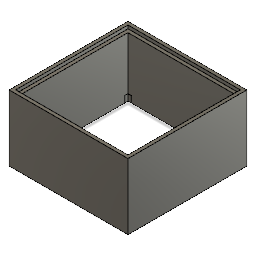
Body-bottom (Autodesk Fusion 360 design; units mm, degrees)
Autodesk Fusion 360 part; units mm, degrees
sketch "Sketch2" plane through (0, 0, 0) normal (0, 1, 0) x (1, 0, 0)
  line L0 (-80, -90) -> (100, -90)
  line L1 (100, -90) -> (100, 90)
  line L2 (100, 90) -> (-80, 90)
  line L3 (-80, 90) -> (-80, -90)
  dimension "d3" = 180
  dimension "d4" = 180
  constraint horizontal L0
  constraint vertical L1
  constraint horizontal L2
  constraint vertical L3
  measures "d3" distance of L0.start L0.end
  measures "d4" distance of L0.start L2.end
extrude "Extrude1" add sketch "Sketch2" along normal blind 100
sketch "Sketch3" plane through (0, 100, 0) normal (0, 1, 0) x (-1, 0, 0)
  line L0 (80, -90) -> (80, 90)
  line L1 (80, 90) -> (-100, 90)
  line L2 (-100, 90) -> (-100, -90)
  line L3 (-100, -90) -> (80, -90)
  line L4 (75, -85) -> (-95, -85)
  line L5 (-95, -85) -> (-95, 85)
  line L6 (-95, 85) -> (75, 85)
  line L7 (75, 85) -> (75, -85)
  constraint horizontal L4
  constraint vertical L5
  constraint horizontal L6
  constraint vertical L7
extrude "Extrude2" cut sketch "Sketch3" against normal blind 5 contours L4 L5 L6 L7
sketch "Sketch4" plane through (0, 95, 0) normal (0, 1, 0) x (-1, 0, 0)
  line L0 (75, 85) -> (-95, 85)
  line L1 (-95, 85) -> (-95, -85)
  line L2 (-95, -85) -> (75, -85)
  line L3 (75, -85) -> (75, 85)
  line L4 (70, 80) -> (-90, 80)
  line L5 (-90, 80) -> (-90, -80)
  line L6 (-90, -80) -> (70, -80)
  line L7 (70, -80) -> (70, 80)
  constraint horizontal L4
  constraint vertical L5
  constraint horizontal L6
  constraint vertical L7
extrude "Extrude3" cut sketch "Sketch4" against normal blind 175 contours L4 L5 L6 L7
sketch "Sketch5" plane through (0, 0, 0) normal (0, -1, 0) x (1, 0, 0)
  line L0 (-70, 80) -> (90, 80)
  line L1 (90, 80) -> (90, -80)
  line L2 (90, -80) -> (-70, -80)
  line L3 (-70, -80) -> (-70, 80)
  line L4 (-80, 90) -> (-80, -90)
  line L5 (-80, -90) -> (100, -90)
  line L6 (100, -90) -> (100, 90)
  line L7 (100, 90) -> (-80, 90)
  line L8 (95, -85) -> (-75, -85)
  line L9 (-75, -85) -> (-75, 85)
  line L10 (-75, 85) -> (95, 85)
  line L11 (95, 85) -> (95, -85)
  point P0 (95, -85)
  point P1 (-75, 85)
  constraint horizontal L8
  constraint vertical L9
  constraint horizontal L10
  constraint vertical L11
  constraint coincident P1 L9.end
  constraint coincident P0 L8.start
extrude "Extrude4" cut sketch "Sketch5" against normal blind 5 contours L8 L9 L10 L11
sketch "Sketch6" plane through (0, 0, 0) normal (0, -1, 0) x (1, 0, 0)
  line L0 (-75, -85) -> (-75, 85)
  line L1 (-75, 85) -> (95, 85)
  line L2 (95, 85) -> (95, -85)
  line L3 (95, -85) -> (-75, -85)
  line L4 (-80, 90) -> (-80, -90)
  line L5 (-80, -90) -> (100, -90)
  line L6 (100, -90) -> (100, 90)
  line L7 (100, 90) -> (-80, 90)
  line L8 (95, -85) -> (85, -85)
  line L9 (85, -85) -> (85, -75)
  line L10 (85, -75) -> (95, -75)
  line L11 (95, -75) -> (95, -85)
  dimension "d13" = 10
  constraint horizontal L8
  constraint vertical L9
  constraint horizontal L10
  constraint vertical L11
  constraint coincident L2.end L3.start
  measures "d13" distance of L2.end L8.end
extrude "Extrude5" cut sketch "Sketch6" against normal blind 10 contours L2 L3 L8 L9 L10 L11
sketch "Sketch7" plane through (0, 5, 0) normal (0, -1, 0) x (1, 0, 0)
  line L0 (90, -75) -> (95, -75)
  line L1 (95, -75) -> (95, 85)
  line L2 (95, 85) -> (-75, 85)
  line L3 (-75, 85) -> (-75, -85)
  line L4 (-75, -85) -> (85, -85)
  line L5 (85, -85) -> (85, -80)
  line L6 (85, -80) -> (-70, -80)
  line L7 (-70, -80) -> (-70, 80)
  line L8 (-70, 80) -> (90, 80)
  line L9 (90, 80) -> (90, -75)
  line L10 (95, 85) -> (85, 85)
  line L11 (85, 85) -> (85, 75)
  line L12 (85, 75) -> (95, 75)
  line L13 (95, 75) -> (95, 85)
  constraint horizontal L10
  constraint vertical L11
  constraint horizontal L12
  constraint vertical L13
  constraint coincident L1.end L2.start
extrude "Extrude6" cut sketch "Sketch7" against normal blind 10 contours L1 L2 L8 L9 L10 L11 L12 L13
sketch "Sketch8" plane through (0, 5, 0) normal (0, -1, 0) x (1, 0, 0)
  line L0 (85, 80) -> (85, 85)
  line L1 (85, 85) -> (-75, 85)
  line L2 (-75, 85) -> (-75, -85)
  line L3 (-75, -85) -> (85, -85)
  line L4 (85, -85) -> (85, -80)
  line L5 (85, -80) -> (-70, -80)
  line L6 (-70, -80) -> (-70, 80)
  line L7 (-70, 80) -> (85, 80)
  line L8 (-75, -85) -> (-65, -85)
  line L9 (-65, -85) -> (-65, -75)
  line L10 (-65, -75) -> (-75, -75)
  line L11 (-75, -75) -> (-75, -85)
  constraint horizontal L8
  constraint vertical L9
  constraint horizontal L10
  constraint vertical L11
  constraint coincident L2.end L3.start
extrude "Extrude7" cut sketch "Sketch8" against normal blind 10 contours L2 L3 L5 L6 L8 L9 L10 L11
sketch "Sketch9" plane through (0, 5, 0) normal (0, -1, 0) x (1, 0, 0)
  line L0 (-75, -75) -> (-70, -75)
  line L1 (-70, -75) -> (-70, 80)
  line L2 (-70, 80) -> (85, 80)
  line L3 (85, 80) -> (85, 85)
  line L4 (85, 85) -> (-75, 85)
  line L5 (-75, 85) -> (-75, -75)
  line L6 (-75, 85) -> (-65, 85)
  line L7 (-65, 85) -> (-65, 75)
  line L8 (-65, 75) -> (-75, 75)
  line L9 (-75, 75) -> (-75, 85)
  constraint horizontal L6
  constraint vertical L7
  constraint horizontal L8
  constraint vertical L9
  constraint coincident L4.end L5.start
extrude "Extrude8" cut sketch "Sketch9" against normal blind 10 contours L1 L2 L4 L5 L6 L7 L8 L9
sketch "Sketch11" plane through (-75, 0, 0) normal (1, 0, 0) x (0, 0, -1)
  line L0 (85, 100) -> (-85, 100)
  line L1 (-85, 100) -> (-85, 95)
  line L2 (-85, 95) -> (85, 95)
  line L3 (85, 95) -> (85, 100)
